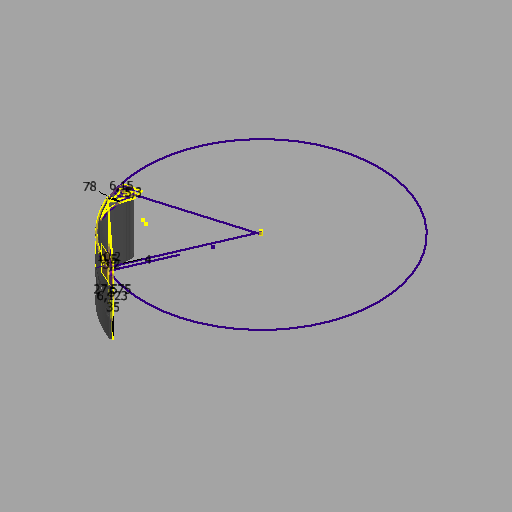
# Autodesk Inventor part: protect_v2.2
Saved by Autodesk Inventor 2023 (Build 270158000, 158)
## iProperties
Created: 2024-10-31
Part Number: protect_v2.2
Material: Типовые
Document SubType Name: Modeling
Designer: Ivan
Density: 0.80427 g/cm^3
Appearance: Типовые
Mass: 79 g
Surface Area: 341.156 cm^2
Volume: 98.2257 cm^3
Author: Ivan
Autodesk Inventor part; units mm, degrees
ref_plane "YZ Plane" through (0, 0, 0) normal (1, 0, 0) x (0, 1, 0)
ref_plane "XZ Plane" through (0, 0, 0) normal (0, 1, 0) x (-1, 0, 0)
ref_plane "XY Plane" through (0, 0, 0) normal (0, 0, 1) x (1, 0, 0)
derived "floor_v2.ipt"
sketch "Эскиз2" plane through (0, 0, 0) normal (0, 1, 0) x (1, 0, 0)
  circle A0 centre (0, 0) radius 107.5
  circle A1 centre (0, 0) radius 104
  line L0 (0, 0) -> (104, 0) construction
  line L1 (0, 0) -> (0, -104) construction
  line L2 (0, 0) -> (-104, 0) construction
  line L3 (0, 0) -> (0, 104) construction
  line L4 (104, 0) -> (0, -104) construction
  line L5 (0, 104) -> (-104, 0) construction
  line L6 (0, -104) -> (-104, 0) construction
  line L7 (104, 0) -> (0, 104) construction
  line L8 (0, 0) -> (-73.539105, -73.539105) construction
  line L9 (0, 0) -> (73.539105, -73.539105) construction
  line L10 (0, 0) -> (73.539105, 73.539105) construction
  line L11 (0, 0) -> (-73.539105, 73.539105) construction
  line L12 (-38.447059, -82.28768) -> (-82.28768, -38.447059)
  line L13 (-38.447059, -82.28768) -> (-48.275844, -92.116464)
  line L14 (-82.28768, -38.447059) -> (-92.116464, -48.275844)
  line L15 (92.116464, -48.275844) -> (82.28768, -38.447059)
  line L16 (82.28768, -38.447059) -> (38.447059, -82.28768)
  line L17 (38.447059, -82.28768) -> (48.275844, -92.116464)
  line L18 (48.275844, 92.116464) -> (38.447059, 82.28768)
  line L19 (38.447059, 82.28768) -> (82.28768, 38.447059)
  line L20 (82.28768, 38.447059) -> (92.116464, 48.275844)
  line L21 (-48.275844, 92.116464) -> (-38.447059, 82.28768)
  line L22 (-38.447059, 82.28768) -> (-82.28768, 38.447059)
  line L23 (-82.28768, 38.447059) -> (-92.116464, 48.275844)
  line L24 (0, -107.5) -> (0, -79.5) construction
  circle A2 centre (0, -116.5) radius 37 construction
  circle A3 centre (0, -127) radius 47.5
  line L25 (0, 107.5) -> (0, 79.5) construction
  circle A4 centre (0, 127) radius 47.5
  line L26 (-92.116464, 48.275844) -> (-94.705096, 50.864475)
  line L27 (-48.275844, 92.116464) -> (-50.864475, 94.705096)
  line L28 (48.275844, 92.116464) -> (50.864475, 94.705096)
  line L29 (92.116464, 48.275844) -> (94.705096, 50.864475)
  line L30 (92.116464, -48.275844) -> (94.705096, -50.864475)
  line L31 (48.275844, -92.116464) -> (50.864475, -94.705096)
  line L32 (-92.116464, -48.275844) -> (-94.705096, -50.864475)
  line L33 (-48.275844, -92.116464) -> (-50.864475, -94.705096)
  point P0 (-52, -52)
  point P1 (-52, 52)
  point P2 (52, 52)
  point P3 (52, -52)
  point P4 (-60.367369, -60.367369)
  point P5 (60.367369, -60.367369)
  point P6 (60.367369, 60.367369)
  point P7 (-60.367369, 60.367369)
  point P8 (-36.989164, -97.199803)
  point P9 (36.989164, -97.199803)
  point P10 (36.989164, 97.199803)
  point P11 (-36.989164, 97.199803)
  point P12 (-39.158681, 100.114173)
  point P13 (-39.158681, -100.114173)
sketch "Эскиз7" plane through (0, 2, 0) normal (0, -1, 0) x (-1, 0, 0)
  circle A0 centre (0, 0) radius 94.2655 construction
  circle A1 centre (-90.348132, 26.892369) radius 1.5
  circle A2 centre (-90.348132, -26.892369) radius 1.5
  circle A3 centre (90.348132, 26.892369) radius 1.5
  circle A4 centre (90.348132, -26.892369) radius 1.5
  line L0 (-92.116464, 48.275844) -> (-82.28768, 38.447059)
  line L1 (-82.28768, -38.447059) -> (-92.116464, -48.275844)
  line L2 (92.116464, -48.275844) -> (82.28768, -38.447059)
  line L3 (82.28768, 38.447059) -> (92.116464, 48.275844)
sketch "Эскиз4" plane through (0, 0, 0) normal (0, 1, 0) x (-1, 0, 0)
  circle A0 centre (0, 0) radius 104
  line L0 (92.116464, 48.275844) -> (82.28768, 38.447059)
  line L1 (82.28768, -38.447059) -> (92.116464, -48.275844)
  circle A1 centre (90.348132, -26.892369) radius 1.5
  circle A2 centre (90.348132, 26.892369) radius 1.5
  arc A3 (82.28768, -38.447059) -> (82.28768, 38.447059) centre (0, 0) ccw
  line L2 (90.348132, 26.892369) -> (0, 0) construction
  line L3 (0, 0) -> (90.348132, -26.892369) construction
  line L4 (90.348132, 26.892369) -> (91.785797, 27.320294) construction
  line L5 (90.348132, -26.892369) -> (91.785797, -27.320294) construction
  arc A4 (91.785797, -27.320294) -> (91.785797, 27.320294) centre (0, 0) ccw
  line L6 (88.524704, 20.317858) -> (93.338618, 21.42273)
  line L7 (88.524704, -20.317858) -> (93.338618, -21.42273)
  dimension "d1" = 6
  dimension "d2" = 6
  constraints: 12 end point, 8 point on circle, 2 centre point, 2 coincident, 2 collinear, 2 point on line, 4 other
  measures "d1" distance from line of L6 L2.start
  measures "d2" distance from line of L7 L3.end
extrude "Выдавливание1" add sketch "Эскиз4" along normal blind 50 contours A0 L1 A3 L7 A4 L6 L0 | A1 | A2
sketch "Эскиз5" plane through (0, 0, 0) normal (0, -1, 0) x (1, 0, 0)
  line L0 (-38.447059, 82.28768) -> (-48.275844, 92.116464)
  line L1 (-48.275844, -92.116464) -> (-38.447059, -82.28768)
  circle A0 centre (0, 0) radius 104
  circle A1 centre (0, 0) radius 107.5
  line L2 (-48.275844, 92.116464) -> (-50.864475, 94.705096)
  line L3 (-48.275844, -92.116464) -> (-50.864475, -94.705096)
  constraints: 4 end point, 2 collinear, 2 point on circle
extrude "Выдавливание2" add sketch "Эскиз2" along normal blind 53.15 and the other way blind 2 contours A4 A1 L27 A0 | A0 L33 A1 A3 | L27 A1 L26 A0 | A0 L32 A1 L33 | L26 A1 L32 A0
ref_plane "РабПлоскость1" through (-36.989164, 0, -97.199803) normal (0.6637718, 0, 0.7479351) x (0, 1, 0)
sketch "Эскиз6" plane through (-36.989164, 0, -97.199803) normal (0.6637718, 0, 0.7479351) x (0, 1, 0)
  line L0 (53.15, -0.311819) -> (-2, -0.311819)
  line L1 (-2, 0) -> (53.15, 0)
  line L2 (25.575, 0) -> (25.575, 67) construction
  circle A0 centre (25.575, 6.1895) radius 1.6 construction
  line L3 (40.575, 6.1895) -> (10.575, 6.1895) construction
  circle A1 centre (40.575, 6.1895) radius 1.6
  circle A2 centre (10.575, 6.1895) radius 1.6
  point P0 (0, 36.852995)
  dimension "d9" = 3.2
  dimension "d10" = 6.1895
  dimension "d68" = 30
  constraints: 4 end point, 3 centre point, 2 coincident, 2 equal radius, 2 midpoint, 1 horizontal, 1 point on line, 1 vertical
  measures "d9" diameter of A0
  measures "d10" distance from line of A0.centre L1
  measures "d68" distance of L3.start L3.end
extrude "Выдавливание3" cut sketch "Эскиз6" against normal blind 10
chamfer "Фаска1" distance 1.4 angle 45 2 edges at (-45.4505, 38.975, -97.4192) (-45.4505, 8.975, -97.4192)
ref_plane "РабПлоскость2" through (0, 0, 0) normal (0, 0, -1) x (0, -1, 0)
sketch "Эскиз8" plane through (0, 50, 0) normal (0, 1, 0) x (1, 0, 0)
  circle A0 centre (-90.348132, -26.892369) radius 1.5
  circle A1 centre (-90.348132, 26.892369) radius 1.5
  point P0 (0, 0)
hole "Отверстие1" at (-90.348132, 50, -26.892369) at (-90.348132, 50, 26.892369) direction (0, -1, 0) diameter 4 depth 7
hole "Отверстие2" at (-90.348132, 0, 26.892369) at (-90.348132, 0, -26.892369) direction (0, 1, 0) diameter 4 depth 7
sketch "Эскиз11" plane through (0, 0, 0) normal (0, 0, -1) x (0, -1, 0)
  line L0 (-87, 137) -> (29, 137)
  line L1 (29, 137) -> (29, -53)
  line L2 (29, -53) -> (-87, -53)
  line L3 (-87, -53) -> (-87, 137)
  point P0 (0, 0)
  constraints: 8 end point, 2 parallel, 1 horizontal, 1 perpendicular
extrude "Выдавливание4" cut sketch "Эскиз11" along normal through all
sketch "Эскиз13" plane through (0, 50, 0) normal (0, 1, 0) x (1, 0, 0)
  line L0 (-95.7655, 0) -> (-104, 0)
  arc A0 (-104, 0) -> (-92.116464, -48.275844) centre (0, 0) ccw
  line L1 (-92.116464, -48.275844) -> (-82.28768, -38.447059)
  arc A1 (-88.524704, -20.317858) -> (-82.28768, -38.447059) centre (0, 0) ccw
  line L2 (-88.524704, -20.317858) -> (-93.338618, -21.42273)
  arc A2 (-95.7655, 0) -> (-93.338618, -21.42273) centre (0, 0) ccw
  circle A3 centre (-90.348132, -26.892369) radius 2
  line L3 (-104, 0) -> (-107.5, 0)
  arc A4 (-107.5, 0) -> (-39.158681, -100.114173) centre (0, 0) ccw
  arc A5 (-36.989164, -97.199803) -> (-39.158681, -100.114173) centre (0, -127) ccw
  arc A6 (-104, 0) -> (-36.989164, -97.199803) centre (0, 0) ccw
  line L4 (-93.338618, -21.42273) -> (-104.775743, -24.047736)
  line L5 (-85.715567, -30.037979) -> (-95.90495, -40.227362)
  dimension "d38" = 5.5
  constraints: 4 end point, 3 point on circle, 1 collinear, 1 parallel
  measures "d38" distance from line of L5 A3.centre
extrude "Выдавливание5" cut sketch "Эскиз13" along normal blind 10 and the other way blind 60 contours A2 L4 A0 L0 | A0 L4 A4 L3 | L5 A1 L1 A0
fillet "Сопряжение1" radius 30 1 edges at (-95.9049, 25, 40.2274)
fillet "Сопряжение3" radius 6.5 1 edges at (-85.7156, 25, 30.038)
sketch "Эскиз14" plane through (0, 50, 0) normal (0, 1, 0) x (1, 0, 0)
  arc A0 (-98.096046, -28.670642) -> (-92.681207, -43.070104) centre (0, 0) ccw
  arc A1 (-86.769762, -32.198557) -> (-83.344076, -62.207435) centre (-59.302516, -44.262983) ccw
  arc A2 (-90.246214, -31.691287) -> (-92.681207, -43.070104) centre (-59.302516, -44.262983) ccw
  circle A3 centre (-90.348132, -26.892369) radius 2
  arc A4 (-95.026491, -27.966129) -> (-90.246214, -31.691287) centre (-90.348132, -26.892369) ccw
  line L0 (-95.026491, -27.966129) -> (-98.096046, -28.670642)
  arc A5 (-86.769762, -32.198557) -> (-86.528575, -27.608774) centre (-92.720999, -29.584598) ccw construction
  line L1 (-88.524704, -20.317858) -> (-101.36444, -23.264786) construction
  arc A6 (-88.524704, -20.317858) -> (-86.528575, -27.608774) centre (0, 0) ccw construction
  dimension "d40" = 4.8
  dimension "d41" = 33.4
  dimension "d42" = 102.2
  constraints: 6 point on circle, 3 centre point, 3 coincident, 2 end point, 1 parallel, 1 point on line
  measures "d40" radius of A4
  measures "d41" radius of A2
  measures "d42" radius of A0
extrude "Выдавливание6" cut sketch "Эскиз14" against normal up to surface (50 mm away) contours L0 A4 A2 A0
fillet "Сопряжение4" radius 0.4 4 edges at (-92.6812, 25, 43.0701) (-98.096, 25, 28.6706) (-95.0265, 25, 27.9661) (-90.2462, 25, 31.6913)
sketch "Эскиз15" plane through (-88.524704, 0, 20.317858) normal (-0.2236999, 0, -0.9746581) x (-0.9746581, 0, 0.2236999)
  line L0 (0, 0) -> (13.17358, 0)
  line L1 (13.17358, -2) -> (13.17358, 0)
  line L2 (13.17358, 50) -> (13.17358, 53.15)
  line L3 (0, 50) -> (13.17358, 50)
  line L4 (0, 0) -> (0, 50)
  line L5 (13.17358, 50) -> (4.321352, 50)
  line L6 (16.67358, 52) -> (13.17358, 52)
  line L7 (13.17358, 52) -> (13.17358, 50)
  line L8 (13.17358, 50) -> (16.67358, 50)
  line L9 (16.67358, 50) -> (16.67358, 52)
  line L10 (16.67358, -2) -> (13.17358, -2)
  line L11 (13.17358, -2) -> (13.17358, 0)
  line L12 (13.17358, 0) -> (16.67358, 0)
  line L13 (16.67358, 0) -> (16.67358, -2)
  line L14 (-90.82642, -13.03) -> (-90.82642, 64.18)
  line L15 (16.67358, -2) -> (13.17358, -2)
  line L16 (16.67358, 53.15) -> (16.67358, -2)
  line L17 (13.17358, 53.15) -> (16.67358, 53.15)
  point P0 (-90.82642, 0)
  point P1 (16.67358, 50)
  point P2 (16.67358, 0)
  constraints: 16 end point, 4 parallel, 2 horizontal, 2 perpendicular
revolve "Вращение1" cut sketch "Эскиз15" angle 13 about axis through (0, -10, 0) along (0, 1, 0) contours L12 L13 L10 L1 | L8 L2 L6 L9 | L6 L2 L17 L16
fillet "Сопряжение5" radius 10 2 edges at (-95.1069, 50, 46.2357) (-95.1069, 0, 46.2357)
ref_plane "РабПлоскость3" through (-93.533038, 53.15, 45.470549) normal (0.6749966, 0, -0.7378208) x (0.7378208, 0, 0.6749966)
sketch "Эскиз16" plane through (-93.533038, 53.15, 45.470549) normal (0.6749966, 0, -0.7378208) x (0.7378208, 0, 0.6749966)
  line L0 (76.636319, 55.15) -> (76.636319, 0)
  line L1 (76.636319, 27.575) -> (21.525, 27.575) construction
  line L2 (58.820914, 22.475) -> (19.314969, 22.475)
  line L3 (19.314969, 22.475) -> (19.314969, 32.675) construction
  line L4 (19.314969, 32.675) -> (58.820914, 32.675)
  line L5 (58.820914, 32.675) -> (58.820914, 22.475) construction
  line L6 (18.814969, 3.15) -> (18.814969, 53.15)
  line L7 (76.636319, 0) -> (0, 0)
  line L8 (76.636319, 55.15) -> (76.636319, 0)
  line L9 (0, 55.15) -> (76.636319, 55.15)
  line L10 (-5.514078, 53.15) -> (18.814969, 53.15)
  line L11 (18.814969, 3.15) -> (18.814969, 53.15)
  line L12 (-6.678765, 3.15) -> (18.814969, 3.15)
  arc A0 (58.820914, 22.475) -> (58.820914, 32.675) centre (58.820914, 27.575) ccw
  arc A1 (19.314969, 32.675) -> (19.314969, 22.475) centre (19.314969, 27.575) ccw
  line L13 (63.920914, 27.575) -> (63.920914, 22.475) construction
  line L14 (70.513536, 10.075) -> (70.513536, 45.075) construction
  line L15 (72.106158, 27.575) -> (68.920914, 27.575) construction
  line L16 (70.513536, 29.175) -> (70.513536, 25.975) construction
  circle A2 centre (70.513536, 10.075) radius 1.6
  circle A3 centre (70.513536, 45.075) radius 1.6
  point P0 (38.31816, 53.15)
  point P1 (68.920914, 27.575)
  point P2 (70.513536, 27.575)
  dimension "d48" = 10.2
  dimension "d49" = 0.5
  dimension "d53" = 5
  dimension "d66" = 35
  dimension "d67" = 3.2
  dimension "d69" = 6.12278
  dimension "d70" = 27.575
  constraints: 18 end point, 6 midpoint, 5 point on circle, 4 centre point, 3 coincident, 3 parallel, 3 point on line, 2 horizontal, 2 perpendicular, 2 vertical, 1 equal radius, 2 other
  measures "d48" distance of L2.end L3.end
  measures "d49" distance from line of point (19.315, 27.575) L6
  measures "d53" distance from line of L13 point (68.921, 27.575)
  measures "d66" distance of L14.start L14.end
  measures "d67" diameter of A2
  measures "d69" distance from line of point (70.514, 27.575) L0
  measures "d70" distance from line of point (70.514, 27.575) L7
sketch "Эскиз17" plane through (0, 50, 0) normal (0, 1, 0) x (1, 0, 0)
  circle A0 centre (-90.348132, -26.892369) radius 2
  circle A1 centre (-90.348132, -26.892369) radius 3.1
  point P0 (0, 0)
  dimension "d54" = 6.2
  constraints: 1 centre point, 1 coincident
  measures "d54" diameter of A1
extrude "Выдавливание8" cut sketch "Эскиз17" against normal through all contours A0 | A1
sketch "Эскиз18" plane through (0, 50, 0) normal (0, 1, 0) x (1, 0, 0)
  point P0 (0, 0)
sketch "Эскиз19" plane through (0, 50, 0) normal (0, 1, 0) x (1, 0, 0)
  line L0 (-104.775743, -24.047736) -> (-88.524704, -20.317858)
  arc A0 (-88.524704, -20.317858) -> (-86.528575, -27.608774) centre (0, 0) ccw
  line L1 (-86.528575, -27.608774) -> (-88.524704, -20.317858) construction
  line L2 (-88.524704, -20.317858) -> (-87.939402, -20.183522)
  line L3 (-86.528575, -27.608774) -> (-85.956471, -27.426232) construction
  arc A1 (-86.769762, -32.198557) -> (-86.528575, -27.608774) centre (-92.720999, -29.584598) ccw
  arc A2 (-86.769762, -32.198557) -> (-85.956471, -27.426232) centre (-92.92307, -28.694458) ccw
  arc A3 (-87.939402, -20.183522) -> (-85.956471, -27.426232) centre (0, 0) ccw
  dimension "d57" = 0.6
  dimension "d58" = 7.08109
  constraints: 6 end point, 4 point on circle, 2 centre point, 2 point on line, 1 coincident, 1 equal length
  measures "d57" distance from line of L1 L2.end
  measures "d58" radius of A2
extrude "Выдавливание9" add sketch "Эскиз19" against normal up to surface (50 mm away)
fillet "Сопряжение6" radius 25 1 edges at (-86.7698, 25, 32.1986)
extrude "Выдавливание10" cut sketch "Эскиз16" against normal through all contours L2 A1 L6 L4 A0 | A1 L6
sketch "Эскиз23" plane through (0, 53.15, 127) normal (0, 1, 0) x (0.8021431, 0, 0.5971318)
  circle A0 centre (-75.835744, 101.872175) radius 107.5
  circle A1 centre (-75.835744, 101.872175) radius 105.65
  arc A2 (-47.46525, 1.816615) -> (-47.46525, -1.816615) centre (0, 0) ccw
  line L0 (-47.46525, -1.816615) -> (-75.835744, 101.872175)
  line L1 (-47.953486, -0.032203) -> (-24.166984, 6.476069)
  line L2 (-47.46525, -1.816615) -> (-38.095824, 0.746972)
  line L3 (-134.323506, 33.170685) -> (-145.521215, 20.017517)
  point P0 (-75.835744, 101.872175)
  point P1 (-105.414511, -1.478425)
  point P2 (-144.321977, 21.426178)
  dimension "d81" = 1.85
  constraints: 6 end point, 3 point on circle, 2 perpendicular, 1 centre point, 1 coincident, 1 point on line, 3 other
  measures "d81" distance between parallel lines of L1 L2
extrude "Выдавливание13" cut sketch "Эскиз23" against normal up to surface (55.15 mm away) contours L3 A1 L0 A0
extrude "Выдавливание14" cut sketch "Эскиз16" against normal through all contours L2 A1 L6 L4 A0 | A1 L6 bodies 1
sketch "Эскиз24" plane through (0, 53.15, 0) normal (0, 1, 0) x (0.7378208, 0, 0.6749966)
  line L0 (38.018899, -98.572237) -> (38.684634, -100.2983)
  arc A0 (38.31816, -96.683601) -> (38.684634, -100.2983) centre (85.724567, -93.703247) ccw
  arc A1 (-38.31816, -96.683601) -> (38.31816, -96.683601) centre (0, 0) ccw
  line L1 (-38.31816, -96.683601) -> (-38.926092, -98.217523)
  arc A2 (-38.926092, -98.217523) -> (38.018899, -98.572237) centre (0, 0) ccw
  arc A3 (38.018899, -98.572237) -> (38.457535, -98.401933) centre (0, 0) ccw
  dimension "d89" = 105.65
  dimension "d90" = 105.65
  constraints: 2 point on circle, 1 centre point, 3 other
  measures "d89" radius of A2
  measures "d90" radius of A3
extrude "Выдавливание15" cut sketch "Эскиз24" against normal up to surface (55.15 mm away) contours A3 A0 L0 bodies 1
sketch "Эскиз25" plane through (0, 50, 0) normal (0, 1, 0) x (1, 0, 0)
  arc A0 (-102.972626, -23.633891) -> (-97.976105, -39.529802) centre (0, 0) ccw
  line L0 (-96.488571, -38.806646) -> (-97.976105, -39.529802)
  arc A1 (-96.488571, -38.806646) -> (-83.344076, -62.207435) centre (0, 0) ccw
  arc A2 (-87.681099, -34.53385) -> (-83.344076, -62.207435) centre (-59.302516, -44.262983) ccw
  arc A3 (-86.546155, -31.772908) -> (-87.681099, -34.53385) centre (-64.03228, -42.64146) ccw
  arc A4 (-86.546155, -31.772908) -> (-85.956471, -27.426232) centre (-92.92307, -28.694458) ccw
  arc A5 (-87.939402, -20.183522) -> (-85.956471, -27.426232) centre (0, 0) ccw
  line L1 (-87.939402, -20.183522) -> (-102.972626, -23.633891)
  circle A6 centre (-90.348132, -26.892369) radius 3.1
  arc A7 (-90.453698, -32.214587) -> (-92.585704, -41.472041) centre (-59.302516, -44.262983) ccw
  arc A8 (-93.349666, -41.60144) -> (-92.585704, -41.472041) centre (-92.984305, -41.438617) ccw
  arc A9 (-97.975705, -29.079223) -> (-93.349666, -41.60144) centre (0, 0) ccw
  arc A10 (-97.681719, -28.575547) -> (-97.975705, -29.079223) centre (-97.592239, -28.96541) ccw
  line L2 (-97.681719, -28.575547) -> (-95.401337, -28.052162)
  arc A11 (-94.930032, -28.322821) -> (-95.401337, -28.052162) centre (-95.311857, -28.442025) ccw
  arc A12 (-94.930032, -28.322821) -> (-90.789948, -31.671993) centre (-90.348132, -26.892369) ccw
  arc A13 (-90.453698, -32.214587) -> (-90.789948, -31.671993) centre (-90.826766, -32.070295) ccw
extrude "Выдавливание16" cut sketch "Эскиз25" against normal blind 0.1 bodies 1
sketch "Эскиз26" plane through (0, 0, 0) normal (0, -1, 0) x (1, 0, 0)
  arc A0 (-92.585704, 41.472041) -> (-90.453698, 32.214587) centre (-59.302516, 44.262983) ccw
  arc A1 (-90.789948, 31.671993) -> (-90.453698, 32.214587) centre (-90.826766, 32.070295) ccw
  arc A2 (-90.789948, 31.671993) -> (-94.930032, 28.322821) centre (-90.348132, 26.892369) ccw
  arc A3 (-95.401337, 28.052162) -> (-94.930032, 28.322821) centre (-95.311857, 28.442025) ccw
  line L0 (-95.401337, 28.052162) -> (-97.681719, 28.575547)
  arc A4 (-97.975705, 29.079223) -> (-97.681719, 28.575547) centre (-97.592239, 28.96541) ccw
  arc A5 (-93.349666, 41.60144) -> (-97.975705, 29.079223) centre (0, 0) ccw
  arc A6 (-92.585704, 41.472041) -> (-93.349666, 41.60144) centre (-92.984305, 41.438617) ccw
  arc A7 (-97.486926, 40.721269) -> (-102.972626, 23.633891) centre (0, 0) ccw
  line L1 (-102.972626, 23.633891) -> (-87.939402, 20.183522)
  arc A8 (-85.956471, 27.426232) -> (-87.939402, 20.183522) centre (0, 0) ccw
  arc A9 (-85.956471, 27.426232) -> (-86.546155, 31.772908) centre (-92.92307, 28.694458) ccw
  arc A10 (-87.681099, 34.53385) -> (-86.546155, 31.772908) centre (-64.03228, 42.64146) ccw
  arc A11 (-83.344076, 62.207435) -> (-87.681099, 34.53385) centre (-59.302516, 44.262983) ccw
  arc A12 (-83.344076, 62.207435) -> (-96.000551, 39.998677) centre (0, 0) ccw
  line L2 (-97.486926, 40.721269) -> (-96.000551, 39.998677)
  circle A13 centre (-90.348132, 26.892369) radius 3.1
extrude "Выдавливание17" cut sketch "Эскиз26" against normal blind 0.1 bodies 1
sketch "Эскиз27" plane through (0, 0.1, 0) normal (0, -1, 0) x (1, 0, 0)
  circle A0 centre (-90.348132, 26.892369) radius 3.1
  circle A1 centre (-90.348132, 26.892369) radius 2.65
  point P0 (0, 0)
  dimension "d97" = 6.2
  dimension "d98" = 5.3
  constraints: 1 centre point, 1 coincident
  measures "d97" diameter of A0
  measures "d98" diameter of A1
extrude "Выдавливание18" add sketch "Эскиз27" against normal up to surface (49.8 mm away) bodies 1
sketch "Эскиз28" plane through (0, 0.1, 0) normal (0, -1, 0) x (1, 0, 0)
  circle A0 centre (-90.348132, 26.892369) radius 2.65
  arc A1 (-101.259529, 30.140177) -> (-101.120209, 23.208731) centre (-90.348132, 26.892369) ccw
  arc A2 (-97.486926, 40.721269) -> (-102.972626, 23.633891) centre (0, 0) ccw
  line L0 (-87.939402, 20.183522) -> (-102.972626, 23.633891)
  point P0 (0, 0)
  constraints: 3 point on circle, 1 centre point, 1 coincident, 1 point on line, 1 tangent
extrude "Выдавливание19" cut sketch "Эскиз28" against normal through all contours A1 L0 A2 bodies 1
sketch "Эскиз29" plane through (0, 49.9, 0) normal (0, 1, 0) x (1, 0, 0)
  circle A0 centre (0, 0) radius 105.65
  arc A1 (-95.016976, -46.191957) -> (-38.046199, -98.561703) centre (0, 0) ccw
  circle A2 centre (-90.348132, -26.892369) radius 2.65
  line L0 (0, 0) -> (-90.348132, -26.892369)
  circle A3 centre (-95.365103, -28.385685) radius 2.65
  line L1 (-95.365103, -28.385685) -> (-101.259529, -30.140177)
  line L2 (-101.259529, -30.140177) -> (-101.853113, -28.14596)
  circle A4 centre (-95.365103, -28.385685) radius 6.15
  arc A5 (-94.930032, -28.322821) -> (-90.789948, -31.671993) centre (-90.348132, -26.892369) ccw
  arc A6 (-90.453698, -32.214587) -> (-90.789948, -31.671993) centre (-90.826766, -32.070295) ccw
  arc A7 (-90.453698, -32.214587) -> (-92.585704, -41.472041) centre (-59.302516, -44.262983) ccw
  arc A8 (-93.349666, -41.60144) -> (-92.585704, -41.472041) centre (-92.984305, -41.438617) ccw
  arc A9 (-97.975705, -29.079223) -> (-93.349666, -41.60144) centre (0, 0) ccw
  arc A10 (-97.681719, -28.575547) -> (-97.975705, -29.079223) centre (-97.592239, -28.96541) ccw
  line L3 (-95.401337, -28.052162) -> (-97.681719, -28.575547)
  arc A11 (-94.930032, -28.322821) -> (-95.401337, -28.052162) centre (-95.311857, -28.442025) ccw
  arc A12 (-101.120209, -23.208731) -> (-101.259529, -30.140177) centre (-90.348132, -26.892369) ccw
  arc A13 (-101.259529, -30.140177) -> (-97.976105, -39.529802) centre (0, 0) ccw
  line L4 (-96.488571, -38.806646) -> (-97.976105, -39.529802)
  arc A14 (-96.488571, -38.806646) -> (-83.344076, -62.207435) centre (0, 0) ccw
  arc A15 (-87.681099, -34.53385) -> (-83.344076, -62.207435) centre (-59.302516, -44.262983) ccw
  arc A16 (-86.546155, -31.772908) -> (-87.681099, -34.53385) centre (-64.03228, -42.64146) ccw
  arc A17 (-86.546155, -31.772908) -> (-85.956471, -27.426232) centre (-92.92307, -28.694458) ccw
  arc A18 (-87.939402, -20.183522) -> (-85.956471, -27.426232) centre (0, 0) ccw
  line L5 (-101.120209, -23.208731) -> (-87.939402, -20.183522)
  circle A19 centre (-90.348132, -26.892369) radius 2.65
  arc A20 (-89.470677, -26.631193) -> (-83.344076, -62.207435) centre (-11.625362, -31.541069) ccw
  point P0 (-90.787161, -24.27899)
  point P1 (-89.286557, -29.320447)
  point P2 (-89.619426, -30.578786)
  point P3 (-89.087957, -40.681436)
  point P4 (-93.633589, -30.391765)
  point P5 (-92.73813, -28.037101)
  point P6 (-92.975105, -27.240953)
  point P7 (-97.974521, -28.84768)
  point P8 (-97.9529, -29.15595)
  point P9 (-97.904978, -29.141685)
  dimension "d104" = 5.3
  dimension "d105" = 6.15
  dimension "d106" = 78
  constraints: 6 end point, 6 point on circle, 4 centre point, 2 point on line, 1 coincident, 1 collinear, 1 concentric, 1 perpendicular
  measures "d104" diameter of A3
  measures "d105" distance from line of L1.start L2
  measures "d106" radius of A20
extrude "Выдавливание20" cut sketch "Эскиз29" against normal through all contours A12 L5 A18 L0 A2 A4 | L0 A18 A17 A16 A15 A20 A4 A2 | A2 A3 A5 A11 L3 A10 bodies 1
extrude "Выдавливание21" add sketch "Эскиз29" against normal up to surface (49.8 mm away) contours L1 A3 A5 A6 A4 A9 | A4 A20 A2 A3 | A4 A6 A7 A8 A9 | A4 A2 A20 | A15 A20 picked at (-89.469933, -28.980959) bodies 1
fillet "Сопряжение8" radius 10 1 edges at (-89.6194, 25, 30.5788)
sketch "Эскиз30" plane through (0, 53.15, 0) normal (0, -1, 0) x (0.7378208, 0, 0.6749966)
  arc A0 (38.457535, 98.401933) -> (38.31816, 96.683601) centre (85.724567, 93.703247) ccw
  arc A1 (38.31816, 96.683601) -> (-38.31816, 96.683601) centre (0, 0) ccw
  arc A2 (38.457535, 98.401933) -> (-38.926092, 98.217523) centre (0, 0) ccw
  spline S0 degree 6 poles (-38.926092, 98.217523) (-39.223994, 98.099457) (-39.537468, 97.973965) (-39.86625, 97.840899) (-40.209922, 97.700153) (-40.567919, 97.551673) (-41.472617, 97.17139) (-42.03541, 96.930703) (-42.621469, 96.675215) (-43.223204, 96.407431) (-43.832485, 96.130567) (-44.441168, 95.848344) knots 0 0 0 0 0 0 0 0.41075913 0.41075913 0.41075913 0.41075913 0.41075913 1 1 1 1 1 1 1
  spline S1 degree 6 poles (-43.832237, 94.311903) (-43.223812, 94.594673) (-42.61474, 94.872017) (-42.013163, 95.140204) (-41.427219, 95.396016) (-40.864504, 95.636953) (-39.959907, 96.017542) (-39.601946, 96.166112) (-39.258298, 96.30692) (-38.929531, 96.440024) (-38.616062, 96.565534) (-38.31816, 96.683601) knots 0 0 0 0 0 0 0 0.58925159 0.58925159 0.58925159 0.58925159 0.58925159 1 1 1 1 1 1 1
  arc A3 (-19.50319, 102.15491) -> (-44.996925, 93.761809) centre (0, 0) ccw
  line L0 (-44.996925, 93.761809) -> (-45.606331, 95.299449)
  arc A4 (-44.441168, 95.848344) -> (-54.366875, 90.587888) centre (0, 0) ccw
  constraints: 2 other
extrude "Выдавливание22" cut sketch "Эскиз30" along normal blind 1.25 bodies 1
sketch "Эскиз31" plane through (0, 51.9, 0) normal (0, 1, 0) x (0.7378208, 0, 0.6749966)
  arc A0 (-40.243725, -97.68503) -> (38.457535, -98.401933) centre (0, 0) ccw
  line L0 (0, 0) -> (34.70438, -99.787417)
  line L1 (38.457535, -98.401933) -> (22.838301, -53.491088)
  point P0 (0, 0)
  dimension "d114" = 4
  constraints: 4 end point, 1 coincident, 1 parallel, 1 point on circle
  measures "d114" distance from line of L0.end L1
ref_plane "РабПлоскость4" through (-41.750552, 51.9, 97.050574) normal (-0.395178, 0, 0.9186046) x (0, -1, 0)
sketch "Эскиз32" plane through (-41.750552, 51.9, 97.050574) normal (-0.395178, 0, 0.9186046) x (0, -1, 0)
  circle A0 centre (17.133479, -0.000354) radius 1.85
  circle A1 centre (35.516667, -0.000234) radius 1.85
  circle A2 centre (17.133479, -0.000354) radius 1.6
  circle A3 centre (35.516667, -0.000234) radius 1.6
  point P0 (51.9, 0)
  dimension "d115" = 3.2
  dimension "d116" = 3.2
  constraints: 2 centre point, 2 coincident
  measures "d115" diameter of A2
  measures "d116" diameter of A3
extrude "Выдавливание23" cut sketch "Эскиз32" against normal blind 10 contours A2 | A3 bodies 1
chamfer "Фаска3" distance 1.4 angle 45 2 edges at (-41.2509, 36.2713, 97.264) (-41.2508, 17.8881, 97.264)
ref_plane "РабПлоскость5" through (-87.216542, 25.575, 59.625475) normal (0.8255234, 0, -0.564368) x (0, 1, 0)
sketch "Эскиз33" plane through (-87.216542, 25.575, 59.625475) normal (0.8255234, 0, -0.564368) x (0, 1, 0)
  spline S0 degree 6 poles (5.075431, 4.316964) (5.037767, 3.92807) (4.966223, 3.548252) (4.863563, 3.181791) (4.733275, 2.832527) (4.57953, 2.50366) (4.297458, 2.002748) (4.179894, 1.816593) (4.055295, 1.639214) (3.924417, 1.470674) (3.78794, 1.310994) (3.423593, 0.922472) (3.188266, 0.706656) (2.942717, 0.512457) (2.688736, 0.339551) (2.427788, 0.187606) (1.816316, -0.113329) (1.461933, -0.24842) (1.100817, -0.349384) (0.735361, -0.416576) (0.367714, -0.450184) (-0.267785, -0.450184) (-0.535555, -0.43236) (-0.802477, -0.396717) (-1.067711, -0.343205) (-1.33037, -0.271728) (-1.811355, -0.105441) (-2.030621, -0.015462) (-2.246697, 0.087885) (-2.458942, 0.204727) (-2.666626, 0.335214) (-2.999952, 0.57298) (-3.128738, 0.672257) (-3.255031, 0.777375) (-3.378576, 0.888378) (-3.499091, 1.005306) (-3.765203, 1.284397) (-3.908774, 1.450261) (-4.046286, 1.625825) (-4.176965, 1.81107) (-4.299948, 2.005924) (-4.584802, 2.514977) (-4.736847, 2.84213) (-4.865682, 3.189359) (-4.967213, 3.553503) (-5.038029, 3.930776) (-5.075431, 4.316964) knots 0 0 0 0 0 0 0 0.12704473 0.12704473 0.12704473 0.12704473 0.12704473 0.20790211 0.20790211 0.20790211 0.20790211 0.20790211 0.33530047 0.33530047 0.33530047 0.33530047 0.33530047 0.50002087 0.50002087 0.50002087 0.50002087 0.50002087 0.6199771 0.6199771 0.6199771 0.6199771 0.6199771 0.72269697 0.72269697 0.72269697 0.72269697 0.72269697 0.7892505 0.7892505 0.7892505 0.7892505 0.7892505 0.87384437 0.87384437 0.87384437 0.87384437 0.87384437 1 1 1 1 1 1 1
  line L0 (5.075431, 4.316964) -> (-5.075431, 4.316964)
  point P0 (-25.575, 0)
  constraints: 1 horizontal alignment, 1 other
extrude "Выдавливание24" cut sketch "Эскиз33" along normal blind 10 bodies 1
sketch "Эскиз34" plane through (0, 0.1, 0) normal (0, -1, 0) x (1, 0, 0)
  line L0 (-97.904978, 29.141685) -> (-97.9529, 29.15595)
  arc A0 (-97.975705, 29.079223) -> (-97.974521, 28.84768) centre (-97.592239, 28.96541) ccw
  arc A1 (-97.904978, 29.141685) -> (-97.974521, 28.84768) centre (-95.365103, 28.385685) ccw
  arc A2 (-97.974521, 28.84768) -> (-97.904978, 29.141685) centre (-95.365103, 28.385685) ccw
  arc A3 (-97.9529, 29.15595) -> (-97.975705, 29.079223) centre (0, 0) ccw
  arc A4 (-97.974521, 28.84768) -> (-97.904978, 29.141685) centre (-95.365103, 28.385685) ccw
  arc A5 (-97.975705, 29.079223) -> (-97.974521, 28.84768) centre (-97.592239, 28.96541) ccw
  arc A6 (-97.9529, 29.15595) -> (-97.975705, 29.079223) centre (0, 0) ccw
  line L1 (-97.904978, 29.141685) -> (-97.9529, 29.15595)
  arc A7 (-89.623616, 32.063019) -> (-89.370752, 29.76055) centre (-79.623839, 31.996102) ccw
  arc A8 (-83.344076, 62.207435) -> (-89.623616, 32.063019) centre (-11.625362, 31.541069) ccw
  arc A9 (-83.344076, 62.207435) -> (-96.000551, 39.998677) centre (0, 0) ccw
  line L2 (-97.486926, 40.721269) -> (-96.000551, 39.998677)
  arc A10 (-97.486926, 40.721269) -> (-101.259529, 30.140177) centre (0, 0) ccw
  arc A11 (-101.259529, 30.140177) -> (-89.370752, 29.76055) centre (-95.365103, 28.385685) ccw
  constraints: 2 point on circle, 1 centre point, 1 concentric
extrude "Выдавливание25" add sketch "Эскиз34" against normal up to surface (49.8 mm away) contours A1 A0 A3 L0 bodies 1
equation "\"d2\" = d1"
equation "\"d90\" = d89"
